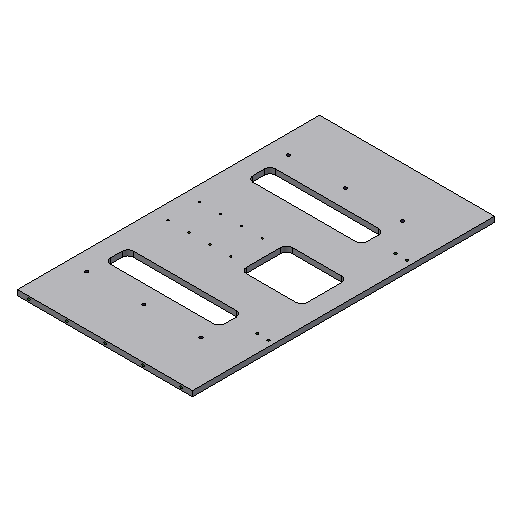
# Autodesk Inventor part: TL20240701-10120CV-001
Saved by Autodesk Inventor 2022.5 (Build 265521000, 521)
## iProperties
Category: FOLLOWER UNIT ASSY
Company: 현대 트랜시스(대유)
RuleStatus: InUse
Created: 2023-04-10
Part Number: TL20240701-10120CV-001
Checked By: 김형민
Engr Approved By: 김시현
User Status: 1 x18
Material: SS400
Description: 0
Document SubType Name: Modeling
Mfg Approved By: 호상태
Designer: 박성규
Stock Number: 001
Mass: 36342.3 g
Surface Area: 8278.95 cm^2
Volume: 4629.59 cm^3
Density: 7.85 g/cm^3
Appearance: Painting-RAL7035
Project: SW PJT
BeforeDocSave0: file://Part Design STD iLogic
DETAIL: Coveryor Assembly
M/C TITLE: CJ 제일제당 협동로봇 포장시스탬 PILOT 장비
PARTS NAME: Bracket
SPECIFICATION: TA20221101-CV200000-015
DocNumber: 221118_Standard_v1
Folder: .\
VDS_Category: 엔지니어링
PLATE_L: 794.000 mm
Detail Description: Processed products
Title: BASE
Subject: SW차종 시트조립라인
Author: 박성규
Revision Number: A
Autodesk Inventor part; units mm, degrees
ref_plane "YZ Plane" through (0, 0, 0) normal (1, 0, 0) x (0, 1, 0)
ref_plane "XZ Plane" through (0, 0, 0) normal (0, 1, 0) x (-1, 0, 0)
ref_plane "XY Plane" through (0, 0, 0) normal (0, 0, 1) x (1, 0, 0)
sketch "스케치9" plane through (0, 0, 0) normal (0, 0, 1) x (1, 0, 0)
  line L0 (-230, 7) -> (230, 7)
  line L1 (230, 7) -> (230, -7)
  line L2 (230, -7) -> (-230, -7)
  line L3 (-230, -7) -> (-230, 7)
  line L4 (-230, 7) -> (230, -7) construction
  line L5 (230, 7) -> (-230, -7) construction
  point P0 (0, 0)
  dimension "d40" = 460
  dimension "d41" = 14
  constraints: 12 end point, 2 midpoint, 2 parallel, 1 horizontal, 1 perpendicular
  measures "d40" distance of L0.start L0.end
  measures "d41" distance of L0.end L1.end
extrude "돌출4" add sketch "스케치9" along normal mid plane 794
sketch "스케치12" plane through (-230, 7, 397) normal (0, 1, 0) x (1, 0, 0)
  line L0 (350, 662) -> (50, 662)
  line L1 (50, 662) -> (50, 132)
  line L2 (50, 132) -> (350, 132)
  line L3 (350, 132) -> (350, 662)
  line L4 (350, 662) -> (50, 132) construction
  line L5 (50, 662) -> (350, 132) construction
  line L6 (460, 0) -> (0, 0) projected
  line L7 (0, 794) -> (460, 794) projected
  line L8 (0, 794) -> (0, 0) projected
  point P0 (200, 397)
  point P1 (200, 397)
  point P2 (200, 397)
  point P3 (200, 132)
  point P4 (200, 662)
  point P5 (185, 662)
  dimension "d66" = 300
  dimension "d97" = 150
  dimension "d135" = 132
  dimension "d143" = 50
  dimension "d144" = 132
  constraints: 12 end point, 6 midpoint, 4 coincident, 2 parallel, 1 horizontal, 1 perpendicular, 1 point on line, 1 vertical alignment
  measures "d66" distance of L1.end L2.end
  measures "d97" distance from line of point (200, 132) L3
  measures "d135" distance between parallel lines of L6 L2
  measures "d143" distance between parallel lines of L1 L8
  measures "d144" distance from line of point (50, 662) L7
hole "구멍4" at (-180, 7, 265) at (120, 7, 265) at (120, 7, -265) at (-180, 7, -265) at (-30, 7, -265) at (-30, 7, 265) direction (0, -1, 0) diameter 8.376 end through all thread size "M10x1.5" class "6H" standard "TS profile"
sketch "스케치13" plane through (0, 0, 397) normal (0, 0, 1) x (1, 0, 0)
  line L0 (-230, -7) -> (230, -7) construction
  line L1 (-230, 7) -> (-230, -7) construction
  line L2 (230, -7) -> (230, 7) construction
  point P0 (0, 0)
  point P1 (-200, 0)
  point P2 (-100, 0)
  point P3 (0, 0)
  point P4 (100, 0)
  point P5 (230, 0)
  point P6 (200, 0)
  dimension "d76" = 30
  dimension "d77" = 7
  dimension "d78" = 100
  dimension "d79" = 100
  dimension "d80" = 100
  dimension "d109" = 100
  dimension "d110" = 30
  constraints: 4 horizontal alignment, 1 midpoint
  measures "d76" distance from line of L1 point (-200, 0)
  measures "d77" distance from line of L0 point (-200, 0)
  measures "d78" distance of point (-100, 0) point (-200, 0)
  measures "d79" distance of point (0, 0) point (-100, 0)
  measures "d80" distance of point (100, 0) point (0, 0)
  measures "d109" distance of point (200, 0) point (100, 0)
  measures "d110" distance from line of L2 point (200, 0)
hole "구멍5" at (-200, 0, 397) at (-100, 0, 397) at (0, 0, 397) at (100, 0, 397) at (200, 0, 397) direction (0, 0, -1) diameter 6.647 depth 22.2 tip angle 118 thread size "M8x1.25" class "6H" standard "TS profile"
sketch "스케치14" plane through (0, 0, -397) normal (0, 0, -1) x (-1, 0, 0)
  circle A0 centre (-100, 0) radius 3.3235 construction
  circle A1 centre (0, 0) radius 3.3235 construction
  circle A2 centre (100, 0) radius 3.3235 construction
  circle A3 centre (200, 0) radius 3.3235 construction
  circle A4 centre (-200, 0) radius 3.3235 construction
  point P0 (0, 0)
  constraints: 5 coincident
hole "구멍6" at (100, 0, -397) at (0, 0, -397) at (-100, 0, -397) at (-200, 0, -397) at (200, 0, -397) direction (0, 0, 1) diameter 6.647 depth 22.2 tip angle 118 thread size "M8x1.25" class "6H" standard "TS profile"
sketch "스케치15" plane through (-230, 7, 397) normal (0, 1, 0) x (1, 0, 0)
  line L0 (460, 794) -> (460, 0) construction
  line L1 (415, 215) -> (445, 215)
  line L2 (445, 215) -> (445, 579)
  line L3 (445, 579) -> (415, 579)
  line L4 (415, 579) -> (415, 215)
  line L5 (415, 215) -> (445, 579) construction
  line L6 (445, 215) -> (415, 579) construction
  point P0 (230, 397)
  point P1 (430, 397)
  point P2 (430, 397)
  dimension "d99" = 364
  dimension "d100" = 30
  dimension "d101" = 15
  constraints: 12 end point, 4 coincident, 3 midpoint, 2 parallel, 1 horizontal, 1 horizontal alignment, 1 perpendicular
  measures "d99" vertical distance of L1.end L3.end
  measures "d100" distance of L2.end L3.end
  measures "d101" distance between parallel lines of L0 L2
hole "구멍7" at (185, 7, 182) at (215, 7, 182) at (215, 7, -182) at (185, 7, -182) direction (0, -1, 0) diameter 6.647 end through all thread size "M8x1.25" class "6H" standard "TS profile"
sketch "스케치16" plane through (-230, 7, 397) normal (0, 1, 0) x (1, 0, 0)
  line L0 (0, 794) -> (460, 794) projected
  line L1 (0, 794) -> (0, 0) projected
  point P0 (230, 397)
  point P1 (95, 438.5)
  point P2 (150, 438.5)
  point P3 (95, 355.5)
  point P4 (150, 355.5)
  point P5 (40, 355.5)
  point P6 (40, 438.5)
  point P7 (95, 355.5)
  point P8 (95, 438.5)
  point P9 (150, 355.5)
  point P10 (150, 438.5)
  point P11 (205, 355.5)
  point P12 (205, 438.5)
  point P13 (0, 397)
  dimension "d148" = 83
  dimension "d149" = 41.5
  dimension "d150" = 40
  dimension "d151" = 55
  dimension "d152" = 55
  dimension "d153" = 55
  constraints: 6 horizontal alignment, 5 vertical alignment, 4 coincident, 1 midpoint
  measures "d148" distance of point (40, 438.5) point (40, 355.5)
  measures "d149" vertical distance of point (0, 397) point (40, 355.5)
  measures "d150" distance from line of L1 point (40, 355.5)
  measures "d151" distance of point (40, 355.5) point (95, 355.5)
  measures "d152" distance of point (150, 355.5) point (95, 355.5)
  measures "d153" distance of point (150, 355.5) point (205, 355.5)
hole "구멍8" at (-80, 7, -41.5) at (-135, 7, -41.5) at (-80, 7, 41.5) at (-135, 7, 41.5) at (-190, 7, 41.5) at (-190, 7, -41.5) at (-25, 7, -41.5) at (-25, 7, 41.5) direction (0, -1, 0) diameter 4.917 end through all thread size "M6x1" class "6H" standard "TS profile"
sketch "스케치18" plane through (-230, 7, 397) normal (0, 1, 0) x (1, 0, 0)
  line L0 (250, 337) -> (410, 337)
  line L1 (410, 337) -> (410, 457)
  line L2 (410, 457) -> (250, 457)
  line L3 (250, 457) -> (250, 337)
  line L4 (250, 337) -> (410, 457) construction
  line L5 (410, 337) -> (250, 457) construction
  line L6 (50, 240) -> (350, 240)
  line L7 (350, 240) -> (350, 180)
  line L8 (350, 180) -> (50, 180)
  line L9 (50, 180) -> (50, 240)
  line L10 (50, 240) -> (350, 180) construction
  line L11 (350, 240) -> (50, 180) construction
  line L12 (50, 554) -> (350, 554)
  line L13 (350, 554) -> (350, 614)
  line L14 (350, 614) -> (50, 614)
  line L15 (50, 614) -> (50, 554)
  line L16 (50, 554) -> (350, 614) construction
  line L17 (350, 554) -> (50, 614) construction
  line L18 (0, 794) -> (0, 0) projected
  line L19 (460, 794) -> (460, 0) projected
  line L20 (460, 0) -> (0, 0) projected
  line L21 (0, 0) -> (0, 794) projected
  line L22 (0, 397) -> (460, 397) construction
  point P0 (200, 210)
  point P1 (330, 397)
  point P2 (200, 210)
  point P3 (200, 584)
  point P4 (200, 584)
  point P5 (330, 397)
  dimension "d126" = 160
  dimension "d138" = 50
  dimension "d140" = 180
  dimension "d141" = 60
  dimension "d145" = 120
  dimension "d146" = 50
  dimension "d147" = 300
  constraints: 38 end point, 10 midpoint, 6 parallel, 3 perpendicular, 2 equal length, 2 horizontal, 1 collinear, 1 point on line, 1 symmetric about line
  measures "d126" distance of L1.end L2.end
  measures "d138" distance between parallel lines of L9 L18
  measures "d140" distance between parallel lines of L8 L20
  measures "d141" distance between parallel lines of L6 L8
  measures "d145" distance of L0.end L1.end
  measures "d146" distance between parallel lines of L1 L19
  measures "d147" distance of L7.end L8.end
extrude "돌출6" cut sketch "스케치18" against normal through all
fillet "모깎기2" radius 15 12 edges at (120, 0, -217) (-180, 0, -217) (-180, 0, -157) (120, 0, -157) (180, 0, 60) (180, 0, -60) (20, 0, -60) (20, 0, 60) (120, 0, 157) (-180, 0, 157) (120, 0, 217) (-180, 0, 217)
equation "\"d97\" = 0.5 * d66"
equation "\"d79\" = d78"
equation "\"d80\" = d79"
equation "\"d109\" = d80"
equation "\"d149\" = 0.5 * d148"
